Autodesk Fusion 360 part; units mm, degrees
note: some values were not read from the file. Chosen so that the rebuilt part matches the saved one: which bodies a step acts on; which face or edge a step refers to; where a step ends. Set by a fixed rule: which sketch regions a step uses.
(part 2 of 2)
sketch "Sketch14" plane through (0, 0, -119.9999) normal (0, 0, -1) x (-1, 0, 0)
  line L0 (-188.975, -0.3374) -> (-188.975, 3.6) construction
  line L1 (-188.975, 3.6) -> (-360, 3.6) construction
  line L2 (-360, 3.6) -> (-360, -0.3374) construction
  line L3 (-360, -0.3374) -> (-188.975, -0.3374) construction
  line L4 (-363, 1.6) -> (-365.75, 1.6) construction
  line L5 (-191.7, 1.6) -> (-194.45, 1.6) construction
  line L6 (-362.35, 1.6) -> (-365.1, 1.6) construction
  line L7 (-362.45, 1.6) -> (-365.2, 1.6) construction
  line L8 (-196.462, 1.6) -> (-199.212, 1.6) construction
  line L9 (-279.55, 1.6) -> (-282.3, 1.6) construction
  line L10 (-277.05, 1.6) -> (-279.8, 1.6) construction
  line L11 (-193.737, 1.6) -> (-360.425, 1.6) construction
  line L12 (-360.425, 1.6) -> (-344.0821, 1.6) construction
  line L13 (-344.0821, 1.6) -> (-342.0821, 1.6) construction
  line L14 (-342.0821, 1.6) -> (-188.975, 1.6) construction
  line L15 (-188.975, 1.6) -> (-365.425, 1.6) construction
  line L16 (-365.425, 1.6) -> (-368.425, 1.6) construction
  line L17 (-365.425, 1.6) -> (-368.425, 1.6) construction
  line L18 (-365.425, 1.6) -> (-193.737, 1.6) construction
  line L19 (-188.975, 3.6) -> (-188.975, -0.3374) construction
  line L20 (-188.365, 1.6) -> (-191.115, 1.6) construction
  line L21 (-62.247, 1.6) -> (-64.997, 1.6) construction
  line L22 (-84.365, 1.6) -> (-87.115, 1.6) construction
  line L23 (-95.865, 1.6) -> (-98.615, 1.6) construction
  line L24 (-3.325, 1.6) -> (-6.075, 1.6) construction
  line L25 (-183.605, 1.6) -> (-186.355, 1.6) construction
  line L26 (-159.58, 1.6) -> (-162.33, 1.6) construction
  line L27 (-3.325, 1.6) -> (-6.075, 1.6) construction
  line L28 (-193.737, 1.6) -> (-3, 1.6) construction
  line L29 (0, 1.6) -> (-3, 1.6) construction
  line L30 (0, 1.6) -> (-3, 1.6) construction
  line L31 (-3, 1.6) -> (-188.975, 1.6) construction
  line L32 (-188.975, 1.6) -> (-55.625, 1.6) construction
  line L33 (-55.625, 1.6) -> (-193.737, 1.6) construction
  line L34 (-26.3429, 1.6) -> (-24.3429, 1.6) construction
  line L35 (-24.3429, 1.6) -> (-8, 1.6) construction
  line L36 (-8, 1.6) -> (-46.1, 1.6) construction
  line L37 (-46.1, 1.6) -> (-26.3429, 1.6) construction
  circle A0 centre (-207.975, -7.7) radius 2.5
  circle A1 centre (-169.975, -7.7) radius 2.5
  circle A2 centre (-207.975, -7.7) radius 2.7
  circle A3 centre (-169.975, -7.7) radius 2.7
  line L38 (-77.725, -5.5) -> (-72.025, -5.5) construction
  line L39 (-72.025, -5.5) -> (-72.025, -8.8)
  line L40 (-72.025, -8.8) -> (-77.725, -8.8) construction
  line L41 (-77.725, -8.8) -> (-77.725, -5.5) construction
  arc A4 (-77.725, -5.5) -> (-77.725, -8.8) centre (-77.725, -7.15) ccw construction
  arc A5 (-72.025, -8.8) -> (-72.025, -5.5) centre (-72.025, -7.15) ccw construction
  line L42 (-79.375, -2.8) -> (-79.375, -8.8) construction
  line L43 (-70.375, -2.8) -> (-70.375, -7.8) construction
  arc A6 (-72.025, -9.2) -> (-72.025, -5.1) centre (-72.025, -7.15) ccw
  line L44 (-77.725, -5.1) -> (-72.025, -5.1)
  arc A7 (-77.725, -5.1) -> (-77.725, -9.2) centre (-77.725, -7.15) ccw
  line L45 (-72.025, -9.2) -> (-77.725, -9.2)
  line L46 (-305.925, -5.5) -> (-300.225, -5.5) construction
  line L47 (-300.225, -5.5) -> (-300.225, -8.8) construction
  line L48 (-300.225, -8.8) -> (-305.925, -8.8) construction
  line L49 (-305.925, -8.8) -> (-305.925, -5.5) construction
  arc A8 (-305.925, -5.5) -> (-305.925, -8.8) centre (-305.925, -7.15) ccw construction
  arc A9 (-300.225, -8.8) -> (-300.225, -5.5) centre (-300.225, -7.15) ccw construction
  line L50 (-307.575, -7.15) -> (-307.575, -10.2748) construction
  arc A10 (-305.925, -5.1) -> (-305.925, -9.2) centre (-305.925, -7.15) ccw
  line L51 (-300.225, -9.2) -> (-305.925, -9.2)
  arc A11 (-300.225, -9.2) -> (-300.225, -5.1) centre (-300.225, -7.15) ccw
  line L52 (-305.925, -5.1) -> (-300.225, -5.1)
  line L53 (-188.975, -3.3374) -> (-360, -3.3374)
  line L54 (-8.425, -3.3374) -> (-188.975, -3.3374)
  line L55 (-360, -10.2748) -> (-188.975, -10.2748)
  line L56 (-188.975, -10.2748) -> (-8.425, -10.2748)
  line L57 (-210.675, -10.2748) -> (-210.675, -5) construction
  line L58 (-210.675, -5) -> (-205.275, -5) construction
  line L59 (-205.275, -5) -> (-205.275, -10.2748) construction
  line L60 (-211.175, -10.2748) -> (-211.175, -4.5)
  line L61 (-211.175, -4.5) -> (-204.775, -4.5)
  line L62 (-204.775, -4.5) -> (-204.775, -10.2748)
  line L63 (-172.675, -10.2748) -> (-172.675, -5) construction
  line L64 (-172.675, -5) -> (-167.275, -5) construction
  line L65 (-167.275, -5) -> (-167.275, -10.2748) construction
  line L66 (-173.175, -10.2748) -> (-173.175, -4.5)
  line L67 (-173.175, -4.5) -> (-166.775, -4.5)
  line L68 (-166.775, -4.5) -> (-166.775, -10.2748)
  line L69 (-298.175, -10.2748) -> (-298.175, -5.1) construction
  line L70 (-307.975, -5.1) -> (-307.975, -10.2748) construction
  line L71 (-307.975, -5.1) -> (-298.175, -5.1) construction
  line L72 (-297.675, -10.2748) -> (-297.675, -4.6)
  line L73 (-308.475, -4.6) -> (-297.675, -4.6)
  line L74 (-308.475, -4.6) -> (-308.475, -10.2748)
  line L75 (-193.737, -8.5374) -> (-8.425, -8.5374)
  line L76 (-8.425, -8.5374) -> (8.626, -8.5374)
  line L77 (-8.425, -8.5374) -> (8.626, -8.5374)
  line L78 (-8.425, -8.5374) -> (-188.975, -8.5374)
  line L79 (-188.975, -8.5374) -> (-8.425, -8.5374)
  line L80 (-8.425, -8.5374) -> (10.626, -8.5374)
  line L81 (-8.425, -8.5374) -> (10.626, -8.5374)
  line L82 (-8.425, -8.5374) -> (-193.737, -8.5374)
  line L83 (-193.737, -8.5374) -> (-360, -8.5374)
  line L84 (-379.051, -8.5374) -> (-360, -8.5374)
  line L85 (-379.051, -8.5374) -> (-360, -8.5374)
  line L86 (-360, -8.5374) -> (-188.975, -8.5374)
  line L87 (-188.975, -8.5374) -> (-360, -8.5374)
  line L88 (-377.051, -8.5374) -> (-360, -8.5374)
  line L89 (-377.051, -8.5374) -> (-360, -8.5374)
  line L90 (-360, -8.5374) -> (-193.737, -8.5374)
  line L91 (-79.775, -10.2748) -> (-79.775, -5.1) construction
  line L92 (-69.975, -10.2748) -> (-69.975, -5.1) construction
  line L93 (-79.775, -5.1) -> (-69.975, -5.1) construction
  line L94 (-80.275, -10.2748) -> (-80.275, -4.6)
  line L95 (-80.275, -4.6) -> (-69.475, -4.6)
  line L96 (-69.475, -10.2748) -> (-69.475, -4.6)
  circle A12 centre (-207.975, -7.7) radius 4
  circle A13 centre (-169.975, -7.7) radius 4
  line L97 (-343.9, 1.6) -> (-357.9, 1.6)
  line L98 (-357.9, 1.6) -> (-343.9, 1.6)
  line L99 (-10.525, 1.6) -> (-24.525, 1.6)
  line L100 (-24.525, 1.6) -> (-10.525, 1.6)
  dimension "d151" = 5
  dimension "d152" = 19
  dimension "d153" = 9.3
  dimension "d154" = 19
  dimension "d155" = 0.2
  dimension "d173" = 118.6
  dimension "d174" = 10.4
  dimension "d175" = 9
  dimension "d178" = 3.3
  dimension "d179" = -0.4
  dimension "d184" = 118.6
  dimension "d187" = -0.4
  dimension "d188" = -0.5
  dimension "d189" = -0.5
  dimension "d190" = -0.5
  dimension "d191" = 0.5
  dimension "d196" = 8
  constraint equal A0 A1
  constraint horizontal A0.centre A1.centre
  constraint concentric A0 A2
  constraint concentric A1 A3
  constraint equal A2 A3
  constraint horizontal L38
  constraint vertical L39
  constraint horizontal L40
  constraint vertical L41
  constraint midpoint L41 A4.centre
  constraint midpoint L39 A5.centre
  constraint vertical L42
  constraint vertical L43
  constraint tangent A5 L43
  constraint tangent A4 L42
  constraint coincident L40.end L41.start
  constraint horizontal L46
  constraint vertical L47
  constraint horizontal L48
  constraint vertical L49
  constraint coincident L48 L49.start
  constraint coincident L49 L48.end
  constraint midpoint L49 A8.centre
  constraint midpoint L47 A9.centre
  constraint vertical L50
  constraint tangent A8 L50
  constraint equal L41 L47
  constraint equal L38 L46
  constraint horizontal A4.centre A9.centre
  constraint coincident L55 L57.start
  constraint perpendicular L55 L57
  constraint perpendicular L57 L58
  constraint coincident L55 L59.end
  constraint perpendicular L55 L59
  constraint tangent A2 L58
  constraint tangent A2 L57
  constraint tangent A2 L59
  constraint coincident L56 L63.start
  constraint perpendicular L56 L63
  constraint perpendicular L63 L64
  constraint coincident L56 L65.end
  constraint perpendicular L56 L65
  constraint tangent A3 L63
  constraint tangent A3 L64
  constraint tangent A3 L65
  constraint coincident L55 L69.start
  constraint perpendicular L55 L69
  constraint tangent A11 L69
  constraint coincident L50.end L55
  constraint coincident L55 L70.end
  constraint perpendicular L55 L70
  constraint tangent A10 L70
  constraint collinear L52 L71
  constraint coincident L56 L91.start
  constraint tangent A7 L91
  constraint perpendicular L56 L91
  constraint vertical L92
  constraint coincident L56 L92.start
  constraint tangent A6 L92
  constraint collinear L44 L93
  constraint concentric A2 A12
  constraint concentric A1 A13
  constraint equal A12 A13
  measures "d151" diameter of A0
  measures "d152" distance of L19 A0.centre
  measures "d153" distance of L15 A0.centre
  measures "d154" distance of L19 A1.centre
  measures "d155" distance of A1 A3
  measures "d173" distance of L19 L43
  measures "d174" distance of L33 L40
  measures "d175" distance of L42 L43
  measures "d178" distance of L38 L40
  measures "d184" distance of L19 L50
  measures "d196" diameter of A12
extrude "Extrude18" cut sketch "Sketch14" against normal blind 20 contours A0 L83 L86 L87 L90 | A0 A2 L83 L86 L87 L90 | A0 L83 L86 L87 L90 | A0 A2 L55 L83 L86 L87 L90 | A2 L55 | A10 A11 L52 L83 L86 L87 L90 | A10 L51 A11 L83 L86 L87 L90 | A3 L56 | A1 A3 L56 L75 L78 L79 L82 | A1 A3 L75 L78 L79 L82 | A1 L75 L78 L79 L82 | A1 L75 L78 L79 L82 | A6 A7 L45 L75 L78 L79 L82 | A6 L44 A7 L75 L78 L79 L82 bodies 3 4 8 9
extrude "Extrude21" cut sketch "Sketch14" against normal blind 10 contours A0 A2 L83 L86 L87 L90 | A2 L60 L61 L62 L83 L86 L87 L90 A12 | L60 L61 A12 | L61 L62 A12 | A10 A11 L52 L72 L73 L74 L83 L86 L87 L90 | A3 L66 L67 L68 L75 L78 L79 L82 A13 | L66 L67 A13 | A1 A3 L75 L78 L79 L82 | L67 L68 A13 | A6 L44 A7 L75 L78 L79 L82 L94 L95 L96 bodies 4 9
extrude "Extrude22" add sketch "Sketch14" against normal up to surface (2.949 mm away) contours A2 L60 L61 L62 L83 L86 L87 L90 A12 | L60 L61 A12 | L61 L62 A12 | A10 A11 L52 L72 L73 L74 L83 L86 L87 L90 | A3 L66 L67 L68 L75 L78 L79 L82 A13 | L66 L67 A13 | L67 L68 A13 | A6 L44 A7 L75 L78 L79 L82 L94 L95 L96 bodies 3 8
extrude "Extrude19" add sketch "Sketch14" along normal up to near side of body 8 contours A3 L56 A13 bodies 8
extrude "Extrude20" add sketch "Sketch14" along normal up to near side of body 3 contours A2 L55 A12 bodies 3
chamfer "Chamfer4" distance 1.42 angle 45 2 edges at (207.975, -11.7, -118.5747) (169.975, -11.7, -118.5747) on bodies 3 8
chamfer "Chamfer5" distance 0.6 angle 45 10 edges at (172.4923, -8.6764, -119.9999) (69.975, -7.15, -119.9999) (74.875, -9.2, -119.9999) (79.775, -7.15, -119.9999) (74.875, -5.1, -119.9999) (303.075, -9.2, -119.9999) (307.975, -7.15, -119.9999) (303.075, -5.1, -119.9999) (298.175, -7.15, -119.9999) (210.4923, -8.6764, -119.9999) on bodies 3 8
move_face "OffsetFaces1" [suppressed]
move_face "OffsetFaces2" [suppressed]
equation "d44 = BPlate2TCase"
equation "d50 = BPlate2BCase"
equation "d55 = Angle"
equation "d65 = ChamferHeight"
equation "BPlate2TCase = PlateThickness + TPlate2TCase"
equation "ChamferHeight = 3 mm"
equation "BPlate2BCase = 20 mm"
equation "Angle = 3 deg"
equation "d71 = -ChamferHeight"
equation "PlateThickness = 1.6 mm"
equation "StripeHeight = 3 mm"
equation "d75 = -ChamferHeight"
equation "d7 = 16 * KeySize"
equation "d8 = 5 * KeySize"
equation "d9 = 2 * KeySize"
equation "d10 = KeySize / 2"
equation "d176 = KeySize"
equation "d180 = KeySize"
equation "d89 = PlateThickness"
equation "d92 = StripeHeight"
equation "d113 = -( TPlate2TCase - 2 mm )"
equation "d117 = PlateThickness"
equation "d119 = 2 mm - Tol"
equation "d120 = -d119"
equation "Tol = 0.2 mm"
equation "d124 = Tol"
equation "d125 = Tol"
equation "d126 = Tol"
equation "d129 = StripeWidth"
equation "d130 = StripeHeight"
equation "d131 = StripeHeight"
equation "StripeWidth = 65 mm"
equation "d135 = -Tol"
equation "TPlate2TCase = 5 mm"
equation "InsertDiam = 2.75 mm"
equation "InsertDepth = 4 mm"
equation "d139 = InsertDiam"
equation "d140 = PlateThickness + InsertDepth"
equation "d142 = 2 mm + 2 * Tol"
equation "d155 = Tol"
equation "PegThickness = 6 mm"
equation "d163 = -Tol"
equation "d164 = -Tol"
equation "d179 = -2 * Tol"
equation "d187 = -2 * Tol"
equation "d196 = d151 + 3 mm"
equation "d203 = Tol"
named bodies: "CaseBR", "CaseTR", "AcrylicR", "PlateR", "Plate L", "CaseBL", "AcrylicL", "CaseTL", "CaseBR (1)"
